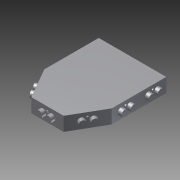
# Autodesk Inventor part: kepala 120 derajat
Saved by Autodesk Inventor 2012 (Build 160160000, 160)
## iProperties
Created: 2013-12-07
Part Number: kepala 120 derajat
Material: Default
Document SubType Name: Modeling
Designer: Irwan Haryanto
Density: 1 g/cm^3
Author: Irwan Haryanto
Autodesk Inventor part; units mm, degrees
ref_plane "YZ Plane" through (0, 0, 0) normal (1, 0, 0) x (0, 1, 0)
ref_plane "XZ Plane" through (0, 0, 0) normal (0, 1, 0) x (-1, 0, 0)
ref_plane "XY Plane" through (0, 0, 0) normal (0, 0, 1) x (1, 0, 0)
sketch "Sketch1" plane through (0, 0, 0) normal (0, 0, 1) x (1, 0, 0)
  line L0 (-41.7418, -140.2167) -> (41.7418, -140.2167)
  line L1 (41.7418, -140.2167) -> (87.255, -219.0478)
  line L2 (87.255, -219.0478) -> (87.255, -359.9816)
  line L3 (87.255, -359.9816) -> (-87.255, -359.9816)
  line L4 (-87.255, -359.9816) -> (-87.255, -219.0478)
  line L5 (-87.255, -219.0478) -> (-41.7418, -140.2167)
  point P0 (0, 0)
  dimension "d0" = 120
  dimension "d1" = 219.7649
  dimension "d2" = 174.51
  dimension "d3" = 120
  dimension "d4" = 150
  dimension "d5" = 150
  dimension "d6" = 91.0263
  dimension "d7" = 91.0263
  dimension "d8" = 83.4837
  dimension "d9" = 140.9338
  dimension "d10" = 140.9338
  constraints: 12 end point, 1 parallel, 1 perpendicular
  measures "d0" angle of L5 L0
  measures "d1" distance between parallel lines of L3 L0
  measures "d2" distance between parallel lines of L2 L4
  measures "d3" angle of L1 L0
  measures "d4" angle of L4 L5
  measures "d5" angle of L2 L1
  measures "d6" distance of L0.end L1.end
  measures "d7" distance of L4.end L0.start
  measures "d8" distance of L0.start L0.end
  measures "d9" distance of L3.end L4.end
  measures "d10" distance of L1.end L2.end
extrude "Extrusion1" add sketch "Sketch1" along normal blind 36
sketch "Sketch2" plane through (-41.7418, -140.2167, 0) normal (0, 1, 0) x (1, 0, 0)
  circle A0 centre (41.7418, -11.1) radius 2.95
  circle A1 centre (61.1168, -25.8) radius 1.5
  circle A2 centre (61.1168, -10.2) radius 1.5
  circle A3 centre (53.4418, -18) radius 8.25
  circle A4 centre (22.3668, -25.8) radius 1.5
  circle A5 centre (30.0418, -18) radius 8.25
  circle A6 centre (22.3668, -10.2) radius 1.5
  point P0 (41.7418, 0)
  dimension "d32" = 0
  dimension "d13" = 16.5
  dimension "d14" = 16.5
  dimension "d15" = 5.9
  dimension "d16" = 3
  dimension "d17" = 7.8
  dimension "d18" = 7.8
  dimension "d19" = 23.4
  dimension "d20" = 7.675
  dimension "d21" = 7.675
  dimension "d22" = 7.675
  dimension "d23" = 7.675
  dimension "d24" = 7.8
  dimension "d25" = 7.8
  dimension "d27" = 6.9
  constraints: 7 centre point
  measures "d13" diameter of A5
  measures "d14" diameter of A3
  measures "d15" diameter of A0
  measures "d16" diameter of A2
  measures "d17" vertical distance of A5.centre A6.centre
  measures "d18" vertical distance of A5.centre A4.centre
  measures "d19" distance of A3.centre A5.centre
  measures "d20" horizontal distance of A5.centre A6.centre
  measures "d21" horizontal distance of A5.centre A4.centre
  measures "d22" horizontal distance of A2.centre A3.centre
  measures "d23" horizontal distance of A1.centre A3.centre
  measures "d24" vertical distance of A3.centre A2.centre
  measures "d25" vertical distance of A3.centre A1.centre
  measures "d27" vertical distance of A0.centre A5.centre
extrude "Extrusion2" add sketch "Sketch2" along normal blind 10 contours A3 | A5
extrude "Extrusion3" add sketch "Sketch2" along normal blind 3 contours A0
sketch "Sketch3" plane through (87.255, -219.0478, 36) normal (0.8660254, 0.5, 0) x (0, 0, -1)
  circle A0 centre (25.8, 26.1382) radius 1.5
  circle A1 centre (18, 33.8132) radius 8.25
  circle A2 centre (10.2, 26.1382) radius 1.5
  circle A3 centre (24.9, 45.5132) radius 2.95
  circle A4 centre (18, 57.2132) radius 8.25
  circle A5 centre (10.2, 64.8882) radius 1.5
  circle A6 centre (25.8, 64.8882) radius 1.5
  point P0 (36, 233.3284)
  point P1 (18, 45.5132)
  point P2 (18, 45.5132)
  dimension "d49" = 16.5
  dimension "d50" = 16.5
  dimension "d51" = 5.9
  dimension "d52" = 3
  dimension "d53" = 7.675
  dimension "d54" = 7.675
  dimension "d55" = 23.4
  dimension "d56" = 7.8
  dimension "d57" = 7.8
  dimension "d58" = 7.8
  dimension "d59" = 7.8
  dimension "d60" = 7.675
  dimension "d61" = 7.675
  dimension "d62" = 11.7
  constraints: 7 centre point
  measures "d49" diameter of A4
  measures "d50" diameter of A1
  measures "d51" diameter of A3
  measures "d52" diameter of A0
  measures "d53" vertical distance of A4.centre A6.centre
  measures "d54" vertical distance of A4.centre A5.centre
  measures "d55" distance of A1.centre A4.centre
  measures "d56" horizontal distance of A4.centre A6.centre
  measures "d57" horizontal distance of A4.centre A5.centre
  measures "d58" horizontal distance of A0.centre A1.centre
  measures "d59" horizontal distance of A2.centre A1.centre
  measures "d60" vertical distance of A1.centre A0.centre
  measures "d61" vertical distance of A1.centre A2.centre
  measures "d62" vertical distance of A3.centre A4.centre
extrude "Extrusion4" add sketch "Sketch3" along normal blind 3 contours A3
extrude "Extrusion5" add sketch "Sketch3" along normal blind 10 contours A1 | A4
sketch "Sketch4" plane through (-41.7418, -140.2167, 0) normal (-0.8660254, 0.5, 0) x (0, 0, 1)
  circle A0 centre (11.1, -45.5132) radius 2.95
  circle A1 centre (25.8, -26.1382) radius 1.5
  circle A2 centre (10.2, -26.1382) radius 1.5
  circle A3 centre (18, -33.8132) radius 8.25
  circle A4 centre (25.8, -64.8882) radius 1.5
  circle A5 centre (18, -57.2132) radius 8.25
  circle A6 centre (10.2, -64.8882) radius 1.5
  point P0 (0, 142.3021)
  point P1 (18, -45.5132)
  point P2 (18, -45.5132)
  dimension "d67" = 16.5
  dimension "d68" = 16.5
  dimension "d69" = 5.9
  dimension "d70" = 3
  dimension "d71" = -7.675
  dimension "d72" = 7.675
  dimension "d73" = 23.4
  dimension "d74" = 7.8
  dimension "d75" = 7.8
  dimension "d76" = 7.8
  dimension "d77" = 7.8
  dimension "d78" = 7.675
  dimension "d79" = 7.675
  dimension "d80" = 6.9
  dimension "d81" = 11.7
  dimension "d82" = 6.9
  constraints: 7 centre point
  measures "d67" diameter of A5
  measures "d68" diameter of A3
  measures "d69" diameter of A0
  measures "d70" diameter of A2
  measures "d71" vertical distance of A5.centre A6.centre
  measures "d72" vertical distance of A5.centre A4.centre
  measures "d73" distance of A3.centre A5.centre
  measures "d74" horizontal distance of A5.centre A6.centre
  measures "d75" horizontal distance of A5.centre A4.centre
  measures "d76" horizontal distance of A2.centre A3.centre
  measures "d77" horizontal distance of A1.centre A3.centre
  measures "d78" vertical distance of A3.centre A2.centre
  measures "d79" vertical distance of A3.centre A1.centre
  measures "d80" horizontal distance of A5.centre A0.centre
  measures "d81" vertical distance of A0.centre A5.centre
  measures "d82" horizontal distance of A3.centre A0.centre
extrude "Extrusion6" add sketch "Sketch4" along normal blind 10 contours A3 | A5
extrude "Extrusion7" add sketch "Sketch4" along normal blind 3 contours A0
sketch "Sketch5" plane through (87.255, -359.9816, 0) normal (1, 0, 0) x (0, 0, -1)
  line L0 (-36, 140.9338) -> (-36, 0) projected
  line L1 (0, 140.9338) -> (0, 0) projected
  line L2 (0, 140.9338) -> (-36, 140.9338) projected
  circle A0 centre (-11.1, 105.7003) radius 2.95
  circle A1 centre (-25.8, 86.3253) radius 1.5
  circle A2 centre (-10.2, 86.3253) radius 1.5
  circle A3 centre (-18, 94.0003) radius 8.25
  circle A4 centre (-25.8, 125.0753) radius 1.5
  circle A5 centre (-18, 117.4003) radius 8.25
  circle A6 centre (-10.2, 125.0753) radius 1.5
  line L3 (-36, 70.4669) -> (0, 70.4669)
  circle A7 centre (-10.2, 54.6085) radius 1.5
  circle A8 centre (-18, 46.9335) radius 8.25
  circle A9 centre (-25.8, 54.6085) radius 1.5
  circle A10 centre (-11.1, 35.2335) radius 2.95
  circle A11 centre (-18, 23.5335) radius 8.25
  circle A12 centre (-25.8, 15.8585) radius 1.5
  circle A13 centre (-10.2, 15.8585) radius 1.5
  point P0 (0, 359.9816)
  point P1 (-18, 105.7003)
  point P2 (-18, 70.4669)
  point P3 (-18, 105.7003)
  point P4 (-18, 35.2335)
  point P5 (-18, 35.2335)
  dimension "d87" = 16.5
  dimension "d88" = 16.5
  dimension "d89" = 5.9
  dimension "d90" = 3
  dimension "d91" = 7.675
  dimension "d92" = 7.675
  dimension "d93" = 23.4
  dimension "d94" = 7.8
  dimension "d95" = 7.8
  dimension "d96" = 7.8
  dimension "d97" = 7.8
  dimension "d98" = 7.675
  dimension "d99" = 7.675
  dimension "d100" = 6.9
  dimension "d101" = 11.7
  dimension "d102" = 6.9
  dimension "d103" = 70.4669
  dimension "d104" = 35.2335
  constraints: 14 centre point, 9 symmetric about line, 2 end point, 2 midpoint, 7 other
  measures "d87" diameter of A5
  measures "d88" diameter of A3
  measures "d89" diameter of A0
  measures "d90" diameter of A2
  measures "d91" vertical distance of A5.centre A6.centre
  measures "d92" vertical distance of A5.centre A4.centre
  measures "d93" distance of A3.centre A5.centre
  measures "d94" horizontal distance of A5.centre A6.centre
  measures "d95" horizontal distance of A5.centre A4.centre
  measures "d96" horizontal distance of A2.centre A3.centre
  measures "d97" horizontal distance of A1.centre A3.centre
  measures "d98" vertical distance of A3.centre A2.centre
  measures "d99" vertical distance of A3.centre A1.centre
  measures "d100" horizontal distance of A5.centre A0.centre
  measures "d101" vertical distance of A0.centre A5.centre
  measures "d102" horizontal distance of A3.centre A0.centre
  measures "d103" distance between parallel lines of L3 L2
  measures "d104" distance from line of L2 point (-18, 105.7)
extrude "Extrusion8" add sketch "Sketch5" along normal blind 3 contours A0 | A10
extrude "Extrusion9" add sketch "Sketch5" along normal blind 10 contours A3 | A5 | A8 | A11
sketch "Sketch6" plane through (-87.255, -359.9816, 0) normal (0, -1, 0) x (1, 0, 0)
  line L0 (174.51, 36) -> (0, 36) projected
  line L1 (174.51, 0) -> (174.51, 36) projected
  line L2 (87.255, 0) -> (87.255, 36)
  circle A0 centre (111.5075, 10.2) radius 1.5
  circle A1 centre (119.1825, 18) radius 8.25
  circle A2 centre (111.5075, 25.8) radius 1.5
  circle A3 centre (130.8825, 11.1) radius 2.95
  circle A4 centre (142.5825, 18) radius 8.25
  circle A5 centre (150.2575, 25.8) radius 1.5
  circle A6 centre (150.2575, 10.2) radius 1.5
  circle A7 centre (43.6275, 11.1) radius 2.95
  circle A8 centre (55.3275, 18) radius 8.25
  circle A9 centre (63.0025, 25.8) radius 1.5
  circle A10 centre (63.0025, 10.2) radius 1.5
  circle A11 centre (24.2525, 10.2) radius 1.5
  circle A12 centre (31.9275, 18) radius 8.25
  circle A13 centre (24.2525, 25.8) radius 1.5
  point P0 (130.8825, 18)
  point P1 (130.8825, 18)
  point P2 (43.6275, 18)
  point P3 (43.6275, 18)
  dimension "d125" = 87.255
  dimension "d126" = 43.6275
  dimension "d127" = 16.5
  dimension "d128" = 16.5
  dimension "d129" = 5.9
  dimension "d130" = 3
  dimension "d131" = -7.8
  dimension "d132" = 7.8
  dimension "d133" = 23.4
  dimension "d134" = 7.675
  dimension "d135" = 7.675
  dimension "d136" = 7.675
  dimension "d137" = 7.675
  dimension "d138" = 7.8
  dimension "d139" = 7.8
  dimension "d140" = 11.7
  dimension "d141" = 6.9
  dimension "d142" = 11.7
  constraints: 14 centre point, 9 symmetric about line, 2 end point, 1 midpoint, 7 other
  measures "d125" distance between parallel lines of L2 L1
  measures "d126" distance from line of point (130.882, 18) L1
  measures "d127" diameter of A4
  measures "d128" diameter of A1
  measures "d129" diameter of A3
  measures "d130" diameter of A0
  measures "d131" vertical distance of A4.centre A6.centre
  measures "d132" vertical distance of A4.centre A5.centre
  measures "d133" distance of A1.centre A4.centre
  measures "d134" horizontal distance of A4.centre A6.centre
  measures "d135" horizontal distance of A4.centre A5.centre
  measures "d136" horizontal distance of A0.centre A1.centre
  measures "d137" horizontal distance of A2.centre A1.centre
  measures "d138" vertical distance of A1.centre A0.centre
  measures "d139" vertical distance of A1.centre A2.centre
  measures "d140" horizontal distance of A4.centre A3.centre
  measures "d141" vertical distance of A3.centre A4.centre
  measures "d142" horizontal distance of A1.centre A3.centre
extrude "Extrusion10" add sketch "Sketch6" along normal blind 10 contours A1 | A4 | A8 | A12
extrude "Extrusion11" add sketch "Sketch6" along normal blind 3 contours A3 | A7
sketch "Sketch7" plane through (-87.255, -359.9816, 0) normal (-1, 0, 0) x (0, 0, 1)
  line L0 (36, 0) -> (36, 140.9338) projected
  line L1 (0, 140.9338) -> (36, 140.9338) projected
  line L2 (0, 0) -> (0, 140.9338) projected
  line L3 (0, 0) -> (36, 0) projected
  point P0 (0, 359.9816)
sketch "Sketch8" plane through (-87.255, -359.9816, 0) normal (-1, 0, 0) x (0, 0, 1)
  line L0 (0, 140.9338) -> (0, 0)
  circle A0 centre (10.2, 54.6085) radius 1.5
  circle A1 centre (18, 46.9335) radius 8.25
  circle A2 centre (25.8, 54.6085) radius 1.5
  circle A3 centre (11.1, 35.2335) radius 2.95
  circle A4 centre (18, 23.5335) radius 8.25
  circle A5 centre (25.8, 15.8585) radius 1.5
  circle A6 centre (10.2, 15.8585) radius 1.5
  circle A7 centre (25.8, 86.3253) radius 1.5
  circle A8 centre (10.2, 86.3253) radius 1.5
  circle A9 centre (18, 94.0003) radius 8.25
  circle A10 centre (11.1, 105.7003) radius 2.95
  circle A11 centre (18, 117.4003) radius 8.25
  circle A12 centre (10.2, 125.0753) radius 1.5
  circle A13 centre (25.8, 125.0753) radius 1.5
  point P0 (0, 359.9816)
  point P1 (0, 359.9816)
  point P2 (18, 35.2335)
  point P3 (18, 70.4669)
  point P4 (18, 35.234)
  point P5 (18, 105.7003)
  point P6 (18, 105.7003)
  point P7 (18, 70.4669)
  dimension "d147" = 16.5
  dimension "d148" = 16.5
  dimension "d149" = 5.9
  dimension "d150" = 3
  dimension "d151" = -7.675
  dimension "d152" = 7.675
  dimension "d153" = 23.4
  dimension "d154" = 7.8
  dimension "d155" = 7.8
  dimension "d156" = 7.8
  dimension "d157" = 7.8
  dimension "d158" = 7.675
  dimension "d159" = 7.675
  dimension "d160" = 6.9
  dimension "d161" = 11.7
  dimension "d162" = 6.9
  constraints: 14 centre point, 2 end point
  measures "d147" diameter of A4
  measures "d148" diameter of A1
  measures "d149" diameter of A3
  measures "d150" diameter of A0
  measures "d151" vertical distance of A4.centre A6.centre
  measures "d152" vertical distance of A4.centre A5.centre
  measures "d153" distance of A1.centre A4.centre
  measures "d154" horizontal distance of A4.centre A6.centre
  measures "d155" horizontal distance of A4.centre A5.centre
  measures "d156" horizontal distance of A0.centre A1.centre
  measures "d157" horizontal distance of A2.centre A1.centre
  measures "d158" vertical distance of A1.centre A0.centre
  measures "d159" vertical distance of A1.centre A2.centre
  measures "d160" horizontal distance of A4.centre A3.centre
  measures "d161" vertical distance of A3.centre A4.centre
  measures "d162" horizontal distance of A1.centre A3.centre
extrude "Extrusion12" add sketch "Sketch8" along normal blind 3 contours A3 | A10
extrude "Extrusion13" add sketch "Sketch8" along normal blind 10 contours A1 | A4 | A9 | A11
body "Solid1"
